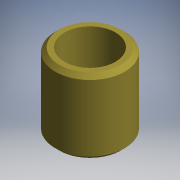
# Autodesk Inventor part: D-3543
Saved by Autodesk Inventor 2017.3 (Build 213256000, 256)
## iProperties
Part Number: D-3543
Material: Generic
Catalog Web Link: www.cadenas.de
Description: Bushing-Original Line - Standard Air Cylinders
Vendor: BIMBA
Document SubType Name: Modeling
Designer: partserver
Manufacturer: BIMBA
Mass: 0.255586 g
Surface Area: 4.87974 cm^2
Volume: 0.255586 cm^3
Density: 1 g/cm^3
Appearance: PSOLRGB-181-165-66
Category: PARTsolutions
Company: BIMBA
Title: D-3543
Author: Cadenas PARTsolutions
Comments: Original Line - Standard Air Cylinders
PSOL_IDENT_0: {$CADENAS_DATA\23d-libs\bimba\bimba_brand\bimba_imperial\bimba_full_line\original_line_cylinders\sta
PSOL_IDENT_1: ndard_air_cylinders\bushing.prj},153 {VTYP=3D},{NB=D-3543},{LINA=D-3543},{NN=Bushing},{DATE=19.01.20
PSOL_IDENT_2: 22 10:19:36},{GEOMDATE=10.09.2012 00:00:00},{VERSION=},{LINEID=30},{WBVAR=},{WBNUMERIC=}  {NB=D-3543
PSOL_IDENT_3: },{LINA=D-3543},{KT=DUMMY},{PN=D-3543},{ID=0.2535},{OD=0.3455},{L=0.3700},{C=0.0200}
NB: D-3543
NN: Bushing
NT: Original Line - Standard Air Cylinders
NBSYN: $PN.
LINA: D-3543
CATALOG: Bimba Products
PN: D-3543
ID: 0.2535
OD: 0.3455
L: 0.37
C: 0.02
SUPPLIER: BIMBA
ARTICLENO: D-3543
BOMINFO: D-3543
CREATOR: CADENAS GmbH
Autodesk Inventor part; units mm, degrees
ref_plane "YZ Plane" through (0, 0, 0) normal (1, 0, 0) x (0, 1, 0)
ref_plane "XZ Plane" through (0, 0, 0) normal (0, 1, 0) x (-1, 0, 0)
ref_plane "XY Plane" through (0, 0, 0) normal (0, 0, 1) x (1, 0, 0)
sketch "Sketch_1" plane through (0, 0, 0) normal (1, 0, 0) x (0, 1, 0)
  line L0 (0, -4.699) -> (0, 4.699)
  line L1 (3.2194, 4.699) -> (3.2194, -4.699)
  line L2 (3.2194, -4.699) -> (3.8799, -4.699)
  line L3 (3.8799, -4.699) -> (4.3879, -4.191)
  line L4 (4.3879, -4.191) -> (4.3879, 4.191)
  line L5 (4.3879, 4.191) -> (3.8799, 4.699)
  line L6 (3.8799, 4.699) -> (3.2194, 4.699)
  constraints: 14 end point
revolve "Revolution1" add sketch "Sketch_1" angle 360 about axis through (0, 0, -4.699) along (0, 0, -1)
ref_plane "bushing_XY" through (0, 0, 0) normal (0, 0, 1) x (1, 0, 0)
ref_plane "bushing_YZ" through (0, 0, 0) normal (1, 0, 0) x (0, 1, 0)
ref_plane "bushing_ZX" through (0, 0, 0) normal (0, 1, 0) x (0, 0, 1)
ref_plane "id1_XY" through (-3.2194, 0, 0) normal (0, 0, 1) x (1, 0, 0)
ref_plane "id1_YZ" through (-3.2194, 0, 0) normal (1, 0, 0) x (0, 1, 0)
ref_plane "id1_ZX" through (-3.2194, 0, 0) normal (0, 1, 0) x (0, 0, 1)
ref_plane "id2_XY" through (3.2194, 0, 0) normal (0, 0, 1) x (1, 0, 0)
ref_plane "id2_YZ" through (3.2194, 0, 0) normal (1, 0, 0) x (0, 1, 0)
ref_plane "id2_ZX" through (3.2194, 0, 0) normal (0, 1, 0) x (0, 0, 1)
ref_plane "id3_XY" through (0, 0, -4.699) normal (0, 0, -1) x (0, 1, 0)
ref_plane "id3_YZ" through (0, 0, -4.699) normal (0, 1, 0) x (1, 0, 0)
ref_plane "id3_ZX" through (0, 0, -4.699) normal (1, 0, 0) x (0, 0, -1)
ref_plane "id4_XY" through (0, 0, 4.699) normal (0, 0, 1) x (0, 1, 0)
ref_plane "id4_YZ" through (0, 0, 4.699) normal (0, 1, 0) x (-1, 0, 0)
ref_plane "id4_ZX" through (0, 0, 4.699) normal (-1, 0, 0) x (0, 0, 1)
body "Solid1"
